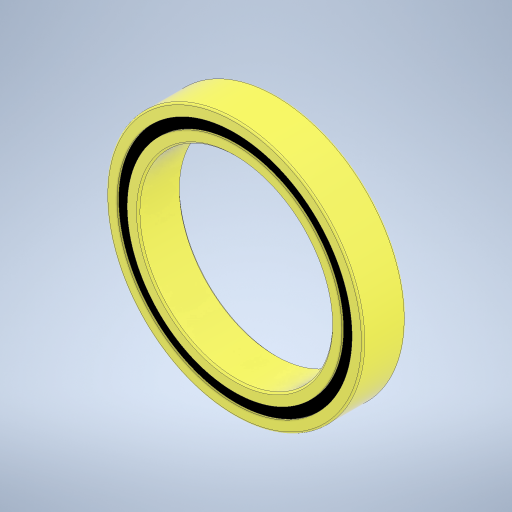
# Autodesk Inventor part: front hub bearing
Saved by Autodesk Inventor 2024 (Build 280153000, 153)
## iProperties
Created: 2023-05-27
Part Number: front hub bearing
Material: Generic
Document SubType Name: Modeling
Designer: _Astitva_Aryan_
Density: 1 g/cm^3
Appearance: Default
Author: _Astitva_Aryan_
Autodesk Inventor part; units mm, degrees
ref_plane "YZ Plane" through (0, 0, 0) normal (1, 0, 0) x (0, 1, 0)
ref_plane "XZ Plane" through (0, 0, 0) normal (0, 1, 0) x (-1, 0, 0)
ref_plane "XY Plane" through (0, 0, 0) normal (0, 0, 1) x (1, 0, 0)
sketch "Sketch1" plane through (0, 0, 0) normal (0, 0, 1) x (1, 0, 0)
  circle A0 centre (0, 0) radius 7.1437
  circle A1 centre (0, 0) radius 9.525
  circle A2 centre (0, 0) radius 7.9566
  circle A3 centre (0, 0) radius 8.7122
  dimension "d0" = 14.2875
  dimension "d1" = 19.05
  dimension "d2" = 0.8128
  dimension "d3" = 0.8128
  constraints: 4 centre point, 2 coincident
  measures "d0" diameter of A0
  measures "d1" diameter of A1
  measures "d2" radial gap between concentric circles of A0 A2
  measures "d3" radial gap between concentric circles of A1 A3
extrude "Extrusion1" add sketch "Sketch1" along normal mid plane 3.175
fillet "Fillet1" radius 0.127 2 edges at (-9.525, 0, 1.5875) (-9.525, 0, -1.5875)
chamfer "Chamfer1" distance 0.127 angle 45 2 edges at (-7.1437, 0, 1.5875) (-7.1437, 0, -1.5875)
sketch "Sketch2" plane through (0, 0, 0) normal (0, 0, 1) x (1, 0, 0)
  circle A0 centre (0, 0) radius 8.7122
  circle A1 centre (0, 0) radius 7.9566
extrude "Extrusion2" add sketch "Sketch2" along normal mid plane 2.921
scale "Scale1" factors (10, 10, 10) then translate (0, 0, 0) bodies 1
body "Solid1"
